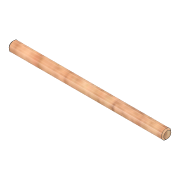
# Autodesk Inventor part: WING_FRONT_TIE
Saved by Autodesk Inventor 2019 (Build 230136000, 136)
## iProperties
Created: 2022-04-02
Part Number: WING_FRONT_TIE
Material: Plywood
Document SubType Name: Modeling
Designer: solyo
Density: 0.746667 g/cm^3
Appearance: Birch - Natural Polished
Mass: 0.279336 g
Surface Area: 3.94112 cm^2
Volume: 0.374111 cm^3
Author: solyo
Autodesk Inventor part; units mm, degrees
ref_plane "YZ Plane" through (0, 0, 0) normal (1, 0, 0) x (0, 1, 0)
ref_plane "XZ Plane" through (0, 0, 0) normal (0, 1, 0) x (-1, 0, 0)
ref_plane "XY Plane" through (0, 0, 0) normal (0, 0, 1) x (1, 0, 0)
sketch "Sketch1" plane through (0, 0, 0) normal (1, 0, 0) x (0, 1, 0)
  circle A0 centre (0, 0) radius 2
  dimension "d0" = 4
  constraints: 1 centre point, 1 coincident
  measures "d0" diameter of A0
extrude "Extrusion1" add sketch "Sketch1" along normal mid plane 64
chamfer "Chamfer1" distance 0.5 angle 45 2 edges at (-32, -2, 0) (32, -2, 0)
equation "\"d1\" = Length"
equation "\"Length\" = 64"
body "Solid1"
